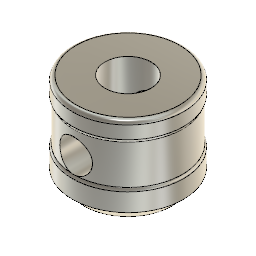
ICMB FUEL INJ MAIN BODY-05 v2 (Autodesk Fusion 360 archive; units mm, degrees)
design "ICBM FUEL INJ -03"
Autodesk Fusion 360 part; units mm, degrees
sketch "Sketch1" plane through (0, 0, 0) normal (0, 0, 1) x (1, 0, 0)
  circle A0 centre (0, 0) radius 4.25
  dimension "d1" = 8.5
  constraint coincident A0.centre origin
  measures "d1" diameter of A0
extrude "Extrude1" add sketch "Sketch1" along normal blind 2.5
sketch "Sketch2" plane through (0, 0, 2.5) normal (0, 0, 1) x (-1, 0, 0)
  circle A0 centre (0, 0) radius 4.25
  circle A1 centre (0, 0) radius 4.15
  dimension "d4" = 8.3
  constraint coincident A0.centre A1.centre
  measures "d4" diameter of A1
extrude "Extrude2" add sketch "Sketch2" along normal blind 3 contours A1
sketch "Sketch3" plane through (0, 0, 5.5) normal (0, 0, 1) x (-1, 0, 0)
  circle A0 centre (0, 0) radius 4.15
  circle A1 centre (0, 0) radius 4.25
  dimension "d7" = 8.5
  constraint coincident A0.centre A1.centre
  measures "d7" diameter of A1
extrude "Extrude3" add sketch "Sketch3" along normal blind 1.5 contours A0 | A1
fillet "Fillet1" radius 0.3 3 edges at (3.9624, 1.5369, 7) (3.9624, 1.5369, 5.5) (-3.9624, -1.5369, 2.5)
chamfer "Chamfer1" distance 0.9 angle 45 1 edges at (-3.9624, -1.5369, 0)
sketch "Sketch4" plane through (0, 0, 7) normal (0, 0, 1) x (-1, 0, 0)
  circle A0 centre (0, 0) radius 3.95
  circle A1 centre (0, 0) radius 1.75
  dimension "d13" = 3.5
  constraint coincident A0.centre A1.centre
  measures "d13" diameter of A1
extrude "Extrude4" cut sketch "Sketch4" against normal blind 6.1 contours A1
sketch "Sketch5" plane through (0, 0, 0.9) normal (0, 0, 1) x (-1, 0, 0)
  circle A0 centre (0, 0) radius 1.75
  circle A1 centre (0, 0) radius 1
  dimension "d16" = 2
  constraint coincident A0.centre A1.centre
  measures "d16" diameter of A1
extrude "Extrude5" cut sketch "Sketch5" against normal blind 5 contours A1
hole "Hole1" at (0, -4.15, 3.7422) direction (0, 1, 0) diameter 2.5 depth 11 tip angle 180
